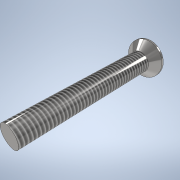
# Autodesk Inventor part: Болт М5х35
Saved by Autodesk Inventor 2021.1 (Build 251245010, 245A)
## iProperties
Created: 2026-05-06
Part Number: Болт М5х35
Material: Типовые
Document SubType Name: Modeling
Designer: Андрей Тарасов
Density: 1 g/cm^3
Appearance: По умолчанию
Author: Андрей Тарасов
Autodesk Inventor part; units mm, degrees
ref_plane "YZ Plane" through (0, 0, 0) normal (1, 0, 0) x (0, 1, 0)
ref_plane "XZ Plane" through (0, 0, 0) normal (0, 1, 0) x (-1, 0, 0)
ref_plane "XY Plane" through (0, 0, 0) normal (0, 0, 1) x (1, 0, 0)
sketch "Эскиз1" plane through (0, 0, 0) normal (0, 0, 1) x (1, 0, 0)
  circle A0 centre (0, 0) radius 4.5
  dimension "d0" = 9
  constraints: 1 centre point, 1 coincident
  measures "d0" diameter of A0
extrude "Выдавливание1" add sketch "Эскиз1" along normal blind 2.5
sketch "Эскиз2" plane through (0, 0, 2.5) normal (0, 0, 1) x (1, 0, 0)
  circle A0 centre (0, 0) radius 2.5
  dimension "d3" = 5
  constraints: 1 centre point, 1 coincident
  measures "d3" diameter of A0
extrude "Выдавливание2" add sketch "Эскиз2" along normal blind 32.5
chamfer "Фаска1" distance 2 angle 45 1 edges at (-4.5, 0, 2.5)
thread "Резьба1" size "M5x0.8" class "6g" standard "ANSI Metric M Profile" full length
sketch "Эскиз3" plane through (0, 0, 0) normal (0, 0, -1) x (-1, 0, 0)
  line L0 (-3, 0.5) -> (3, 0.5)
  line L1 (3, 0.5) -> (3, -0.5)
  line L2 (3, -0.5) -> (-3, -0.5)
  line L3 (-3, -0.5) -> (-3, 0.5)
  line L4 (-0.5, 3) -> (0.5, 3)
  line L5 (0.5, 3) -> (0.5, -3)
  line L6 (0.5, -3) -> (-0.5, -3)
  line L7 (-0.5, -3) -> (-0.5, 3)
  line L8 (0, 3) -> (0, -3) construction
  line L9 (-3, 0) -> (3, 0) construction
  point P0 (0, 0)
  point P1 (0, 0)
  point P2 (-0.5, 0.5)
  point P3 (-0.5, -0.5)
  point P4 (0.5, 0.5)
  point P5 (0.5, -0.5)
  dimension "d12" = 1
  dimension "d13" = 6
  constraints: 20 end point, 6 midpoint, 4 parallel, 4 perpendicular, 2 horizontal, 1 coincident
  measures "d12" distance of L4.start L4.end
  measures "d13" distance of L6.end L4.start
extrude "Выдавливание3" cut sketch "Эскиз3" against normal blind 1
